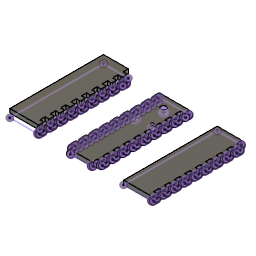
Motor Box (Autodesk Fusion 360 design; units mm, degrees)
part number: 2026-02-17-19-54-44-012
Autodesk Fusion 360 part; units mm, degrees
sketch "Sketch1" plane through (0, 0, 0) normal (0, 0, 1) x (1, 0, 0)
  line L0 (11.75, 48.5) -> (-11.75, 48.5)
  line L1 (-11.75, -48.5) -> (11.75, -48.5)
  line L2 (11.75, -48.5) -> (11.75, 48.5) construction
  line L3 (11.75, 48.5) -> (-11.75, -48.5) construction
  line L4 (-11.75, 48.5) -> (11.75, -48.5) construction
  line L5 (0, 48.5) -> (0, 37.3) construction
  circle A0 centre (0, 37.3) radius 2.7
  line L6 (1.85, 33.3) -> (-1.85, 33.3)
  line L7 (-1.85, 33.3) -> (-1.85, 41.3)
  line L8 (-1.85, 41.3) -> (1.85, 41.3)
  line L9 (1.85, 41.3) -> (1.85, 33.3)
  line L10 (1.85, 33.3) -> (-1.85, 41.3) construction
  line L11 (-1.85, 33.3) -> (1.85, 41.3) construction
  line L12 (0, 48.5) -> (0, 16.7) construction
  line L13 (0, 16.7) -> (8.75, 16.7) construction
  circle A1 centre (8.75, 16.7) radius 1.5
  circle A2 centre (-8.75, 16.7) radius 1.5
  line L14 (11.75, 48.5) -> (15.95, 48.5)
  line L15 (15.95, 48.5) -> (15.95, 43.1111)
  line L16 (15.95, 43.1111) -> (11.75, 43.1111)
  line L17 (11.75, 43.1111) -> (11.75, 37.7222)
  line L18 (11.75, 37.7222) -> (15.95, 37.7222)
  line L19 (15.95, 37.7222) -> (15.95, 32.3333)
  line L20 (15.95, 32.3333) -> (11.75, 32.3333)
  line L21 (11.75, 32.3333) -> (11.75, 26.9444)
  line L22 (11.75, 26.9444) -> (15.95, 26.9444)
  line L23 (15.95, 26.9444) -> (15.95, 21.5556)
  line L24 (15.95, 21.5556) -> (11.75, 21.5556)
  line L25 (11.75, 21.5556) -> (11.75, 16.1667)
  line L26 (11.75, 16.1667) -> (15.95, 16.1667)
  line L27 (15.95, 16.1667) -> (15.95, 10.7778)
  line L28 (15.95, 10.7778) -> (11.75, 10.7778)
  line L29 (11.75, 10.7778) -> (11.75, 5.3889)
  line L30 (11.75, 5.3889) -> (15.95, 5.3889)
  line L31 (15.95, 5.3889) -> (15.95, 0)
  line L32 (15.95, 0) -> (11.75, 0)
  line L33 (11.75, 0) -> (11.75, -5.3889)
  line L34 (11.75, -5.3889) -> (15.95, -5.3889)
  line L35 (15.95, -5.3889) -> (15.95, -10.7778)
  line L36 (15.95, -10.7778) -> (11.75, -10.7778)
  line L37 (11.75, -10.7778) -> (11.75, -16.1667)
  line L38 (11.75, -16.1667) -> (15.95, -16.1667)
  line L39 (15.95, -16.1667) -> (15.95, -21.5556)
  line L40 (15.95, -21.5556) -> (11.75, -21.5556)
  line L41 (11.75, -21.5556) -> (11.75, -26.9444)
  line L42 (11.75, -26.9444) -> (15.95, -26.9444)
  line L43 (15.95, -26.9444) -> (15.95, -32.3333)
  line L44 (15.95, -32.3333) -> (11.75, -32.3333)
  line L45 (11.75, -32.3333) -> (11.75, -37.7222)
  line L46 (11.75, -37.7222) -> (15.95, -37.7222)
  line L47 (15.95, -37.7222) -> (15.95, -43.1111)
  line L48 (15.95, -43.1111) -> (11.75, -43.1111)
  line L49 (11.75, -43.1111) -> (11.75, -48.5)
  line L50 (-15.95, 0) -> (-11.75, 0)
  line L51 (-15.95, 32.3333) -> (-11.75, 32.3333)
  line L52 (-15.95, -10.7778) -> (-11.75, -10.7778)
  line L53 (-15.95, 21.5556) -> (-11.75, 21.5556)
  line L54 (-11.75, 26.9444) -> (-15.95, 26.9444)
  line L55 (-15.95, -43.1111) -> (-11.75, -43.1111)
  line L56 (-15.95, -21.5556) -> (-11.75, -21.5556)
  line L57 (-15.95, -32.3333) -> (-11.75, -32.3333)
  line L58 (-11.75, -32.3333) -> (-11.75, -37.7222)
  line L59 (-15.95, 10.7778) -> (-11.75, 10.7778)
  line L60 (-11.75, 43.1111) -> (-11.75, 37.7222)
  line L61 (-15.95, 5.3889) -> (-15.95, 0)
  line L62 (-11.75, 10.7778) -> (-11.75, 5.3889)
  line L63 (-11.75, -48.5) -> (-11.75, 48.5) construction
  line L64 (-15.95, -16.1667) -> (-15.95, -21.5556)
  line L65 (-11.75, 21.5556) -> (-11.75, 16.1667)
  line L66 (-15.95, 48.5) -> (-15.95, 43.1111)
  line L67 (-15.95, 26.9444) -> (-15.95, 21.5556)
  line L68 (-15.95, -26.9444) -> (-15.95, -32.3333)
  line L69 (-11.75, 5.3889) -> (-15.95, 5.3889)
  line L70 (-11.75, -43.1111) -> (-11.75, -48.5)
  line L71 (-15.95, 16.1667) -> (-15.95, 10.7778)
  line L72 (-15.95, 37.7222) -> (-15.95, 32.3333)
  line L73 (-11.75, -26.9444) -> (-15.95, -26.9444)
  line L74 (-11.75, 32.3333) -> (-11.75, 26.9444)
  line L75 (-11.75, -5.3889) -> (-15.95, -5.3889)
  line L76 (-11.75, -10.7778) -> (-11.75, -16.1667)
  line L77 (-15.95, -37.7222) -> (-15.95, -43.1111)
  line L78 (-15.95, 43.1111) -> (-11.75, 43.1111)
  line L79 (-11.75, 16.1667) -> (-15.95, 16.1667)
  line L80 (-11.75, 0) -> (-11.75, -5.3889)
  line L81 (-15.95, -5.3889) -> (-15.95, -10.7778)
  line L82 (-11.75, -16.1667) -> (-15.95, -16.1667)
  line L83 (-11.75, -21.5556) -> (-11.75, -26.9444)
  line L84 (-11.75, -37.7222) -> (-15.95, -37.7222)
  line L85 (-11.75, 48.5) -> (-15.95, 48.5)
  line L86 (-11.75, 37.7222) -> (-15.95, 37.7222)
  point P0 (0, 37.3)
  dimension "d1" = 23.5
  dimension "d2" = 97
  dimension "d3" = 11.2
  dimension "d4" = 5.4
  dimension "d5" = 3.7
  dimension "d6" = 8
  dimension "d7" = 31.8
  dimension "d8" = 8.75
  dimension "d9" = 3
  dimension "d14" = 4.2
  dimension "d15" = 5.3889
  dimension "d16" = 5.3889
  dimension "d19" = 0
  dimension "d20" = -10.7778
  constraint horizontal L0
  constraint parallel L0 L1
  constraint coincident L3 origin
  constraint coincident L4 origin
  constraint midpoint L0 L5.start
  constraint perpendicular L0 L5
  constraint coincident P0 L5.end
  constraint horizontal L6
  constraint perpendicular L6 L7
  constraint parallel L6 L8
  constraint parallel L7 L9
  constraint coincident L10 P0
  constraint coincident L11 P0
  constraint perpendicular L6 L12
  constraint perpendicular L12 L13
  constraint coincident L13.end A1.centre
  constraint symmetric L12 A1 A2
  constraint horizontal L14
  constraint vertical L15
  constraint horizontal L16
  constraint perpendicular L16 L17
  constraint symmetric L0.start L12 L0.end
  constraint symmetric L1.end L12 L1.start
  constraint symmetric L12 L14.end L66.start
  constraint symmetric L12 L15.end L66.end
  constraint symmetric L12 L16.end L60.start
  constraint symmetric L12 L17.end L60.end
  constraint symmetric L12 L18.end L72.start
  constraint symmetric L12 L19.end L51.start
  constraint symmetric L12 L20.end L51.end
  constraint symmetric L12 L21.end L54.start
  constraint symmetric L12 L22.end L54.end
  constraint symmetric L12 L23.end L53.start
  constraint symmetric L12 L24.end L53.end
  constraint symmetric L12 L25.end L65.end
  constraint symmetric L12 L26.end L71.start
  constraint symmetric L12 L27.end L59.start
  constraint symmetric L12 L28.end L59.end
  constraint symmetric L12 L29.end L62.end
  constraint symmetric L12 L30.end L61.start
  constraint symmetric L12 L31.end L50.start
  constraint symmetric L12 L32.end L50.end
  constraint symmetric L12 L33.end L75.start
  constraint symmetric L12 L34.end L75.end
  constraint symmetric L12 L35.end L52.start
  constraint symmetric L12 L36.end L52.end
  constraint symmetric L12 L37.end L76.end
  constraint symmetric L12 L38.end L64.start
  constraint symmetric L12 L39.end L56.start
  constraint symmetric L12 L40.end L56.end
  constraint symmetric L12 L41.end L73.start
  constraint symmetric L12 L42.end L68.start
  constraint symmetric L12 L43.end L57.start
  constraint symmetric L12 L44.end L57.end
  constraint symmetric L12 L45.end L58.end
  constraint symmetric L12 L46.end L77.start
  constraint symmetric L12 L47.end L55.start
  constraint symmetric L12 L48.end L55.end
  constraint symmetric L12 L1.end L1.start
  constraint coincident L17.end L18.start
  measures "d1" distance of L1.start L1.end
  measures "d2" distance of L0.end L1.start
  measures "d3" distance of L5.start P0
  measures "d4" diameter of A0
  measures "d5" distance of L7.end L8.end
  measures "d6" distance of L6.end L7.end
  measures "d7" distance of L5.start L12.end
  measures "d8" distance of L12.end L13.end
  measures "d9" diameter of A1
  measures "d14" distance of L0.start L14.end
  measures "d15" distance of L0.start L16.end
  measures "d16" distance of L16.end L17.end
extrude "Extrude1" add sketch "Sketch1" along normal blind 4.2 contours L0 L1 L14 L15 L16 L17 L18 L19 L20 L21 L22 L23 L24 L25 L26 L27 L28 L29 L30 L31 L32 L33 L34 L35 L36 L37 L38 L39 L40 L41 L42 L43 L44 L45 L46 L47 L48 L49 L50 L51 L52 L53 L54 L55 L56 L57 L58 L59 L60 L61 L62 L64 L65 L66 L67 L68 L69 L70 L71 L72 L73 L74 L75 L76 L77 L78 L79 L80 L81 L82 L83 L84 L85 L86 | A0 L7 L8 L9 | A0 L6 L7 L9 makes body 1
sketch "Sketch2" plane through (15.95, 0, 0) normal (1, 0, 0) x (0, 1, 0)
  line L0 (-48.5, 0) -> (48.5, 0) construction
  line L1 (48.5, 0) -> (48.5, 30)
  line L2 (48.5, 30) -> (-48.5, 30)
  line L3 (-48.5, 30) -> (-48.5, 0)
  line L4 (-37.7222, 0) -> (-37.7222, 4.2)
  line L5 (-37.7222, 4.2) -> (-43.1111, 4.2)
  line L6 (-43.1111, 4.2) -> (-43.1111, 0)
  line L7 (-48.5, 0) -> (-43.1111, 0)
  line L8 (-37.7222, 0) -> (-32.3333, 0)
  line L9 (-32.3333, 4.2) -> (-32.3333, 0)
  line L10 (-26.9444, 4.2) -> (-32.3333, 4.2)
  line L11 (-26.9444, 0) -> (-26.9444, 4.2)
  line L12 (-26.9444, 0) -> (-21.5556, 0)
  line L13 (-21.5556, 4.2) -> (-21.5556, 0)
  line L14 (-16.1667, 4.2) -> (-21.5556, 4.2)
  line L15 (-16.1667, 0) -> (-16.1667, 4.2)
  line L16 (-16.1667, 0) -> (-10.7778, 0)
  line L17 (-10.7778, 4.2) -> (-10.7778, 0)
  line L18 (-5.3889, 4.2) -> (-10.7778, 4.2)
  line L19 (-5.3889, 0) -> (-5.3889, 4.2)
  line L20 (-5.3889, 0) -> (0, 0)
  line L21 (0, 4.2) -> (0, 0)
  line L22 (5.3889, 4.2) -> (0, 4.2)
  line L23 (5.3889, 0) -> (5.3889, 4.2)
  line L24 (5.3889, 0) -> (10.7778, 0)
  line L25 (10.7778, 4.2) -> (10.7778, 0)
  line L26 (16.1667, 4.2) -> (10.7778, 4.2)
  line L27 (16.1667, 0) -> (16.1667, 4.2)
  line L28 (16.1667, 0) -> (21.5556, 0)
  line L29 (21.5556, 4.2) -> (21.5556, 0)
  line L30 (26.9444, 4.2) -> (21.5556, 4.2)
  line L31 (26.9444, 0) -> (26.9444, 4.2)
  line L32 (26.9444, 0) -> (32.3333, 0)
  line L33 (32.3333, 4.2) -> (32.3333, 0)
  line L34 (37.7222, 4.2) -> (32.3333, 4.2)
  line L35 (37.7222, 0) -> (37.7222, 4.2)
  line L36 (37.7222, 0) -> (43.1111, 0)
  line L37 (43.1111, 4.2) -> (43.1111, 0)
  line L38 (48.5, 4.2) -> (43.1111, 4.2)
  line L39 (48.5, 0) -> (48.5, 4.2)
  point P0 (-48.5, 0)
  point P1 (-43.1111, 0)
  dimension "d23" = 97
  dimension "d24" = 30
  dimension "d25" = 5.3889
  dimension "d26" = 4.2
  dimension "d29" = 10.7778
  dimension "d30" = 0
  constraint horizontal L0
  constraint vertical L1
  constraint horizontal L2
  constraint vertical L3
  constraint coincident P0 L0.start
  constraint vertical L4
  constraint horizontal L5
  constraint vertical L6
  constraint coincident P1 L6.end
  measures "d23" distance of P0 L0.end
  measures "d24" distance of P0 L2.end
  measures "d25" distance of P1 L4.start
  measures "d26" distance of P1 L5.end
extrude "Extrude2" add sketch "Sketch2" against normal blind 4.2 separate body makes body 2
mirror "Mirror1" about plane through (0, 0, 0) normal (1, 0, 0) of bodies 2 makes body 3
move_body "Move1" bodies 3 to x (1, 0, 0) y (0, 1, 0) z (0, 0, 1) at (-29.0338, -1.4815, 0)
move_body "Move2" bodies 2 to x (1, 0, 0) y (0, 1, 0) z (0, 0, 1) at (32.2243, 4.8146, 0)
fillet "Fillet1" radius 1 38 edges at (-15.95, 48.5, 2.1) (-15.95, 43.1111, 2.1) (-15.95, 37.7222, 2.1) (-15.95, 32.3333, 2.1) (-15.95, 26.9444, 2.1) (-15.95, 21.5556, 2.1) (-15.95, 16.1667, 2.1) (-15.95, 10.7778, 2.1) (-15.95, 5.3889, 2.1) (-15.95, 0, 2.1) (-15.95, -5.3889, 2.1) (-15.95, -10.7778, 2.1) (-15.95, -16.1667, 2.1) (-15.95, -21.5556, 2.1) (-15.95, -26.9444, 2.1) (-15.95, -32.3333, 2.1) (-15.95, -37.7222, 2.1) (-15.95, -43.1111, 2.1) (15.95, -43.1111, 2.1) (15.95, -37.7222, 2.1) (15.95, -32.3333, 2.1) (15.95, -26.9444, 2.1) (15.95, -21.5556, 2.1) (15.95, -16.1667, 2.1) (15.95, -10.7778, 2.1) (15.95, -5.3889, 2.1) (11.75, -48.5, 2.1) (-11.75, -48.5, 2.1) (15.95, 0, 2.1) (15.95, 5.3889, 2.1) (15.95, 10.7778, 2.1) (15.95, 16.1667, 2.1) (15.95, 21.5556, 2.1) (15.95, 26.9444, 2.1) (15.95, 32.3333, 2.1) (15.95, 37.7222, 2.1) (15.95, 43.1111, 2.1) (15.95, 48.5, 2.1) on bodies 1
fillet "Fillet2" radius 1 19 edges at (46.0743, -43.6854, 0) (46.0743, -38.2965, 0) (46.0743, -32.9076, 0) (46.0743, -27.5187, 0) (46.0743, -22.1299, 0) (46.0743, -16.741, 0) (46.0743, -11.3521, 0) (46.0743, -5.9632, 0) (46.0743, -0.5743, 0) (46.0743, 4.8146, 0) (46.0743, 10.2035, 0) (46.0743, 15.5924, 0) (46.0743, 20.9813, 0) (46.0743, 26.3701, 0) (46.0743, 31.759, 0) (46.0743, 37.1479, 0) (46.0743, 42.5368, 0) (46.0743, 47.9257, 0) (46.0743, 53.3146, 4.2) on bodies 2
fillet "Fillet3" radius 1 18 edges at (-42.8838, -49.9815, 0) (-42.8838, -44.5926, 0) (-42.8838, -39.2037, 0) (-42.8838, -33.8149, 0) (-42.8838, -28.426, 0) (-42.8838, -23.0371, 0) (-42.8838, -17.6482, 0) (-42.8838, -12.2593, 0) (-42.8838, -6.8704, 0) (-42.8838, -1.4815, 0) (-42.8838, 3.9074, 0) (-42.8838, 9.2963, 0) (-42.8838, 14.6851, 0) (-42.8838, 20.074, 0) (-42.8838, 25.4629, 0) (-42.8838, 30.8518, 0) (-42.8838, 36.2407, 0) (-42.8838, 41.6296, 0) on bodies 3
move_body "Move3" bodies 3 to x (0, 0, 1) y (0, 1, 0) z (-1, 0, 0) at (-24.4783, 0, 65.4894)
move_body "Move4" bodies 3 to x (1, 0, 0) y (0, 1, 0) z (0, 0, 1) at (39.4783, 1.4815, -24.7055)
move_body "Move5" bodies 3 to x (1, 0, 0) y (0, 1, 0) z (0, 0, 1) at (-45.6208, -9.5411, 0)
move_body "Move6" bodies 2 to x (0, 0, 1) y (0, 1, 0) z (-1, 0, 0) at (69.5265, 0, -18.4221)
move_body "Move7" bodies 2 to x (1, 0, 0) y (0, 1, 0) z (0, 0, 1) at (-54.5265, -4.8146, -29.7522)
move_body "Move8" bodies 2 to x (1, 0, 0) y (0, 1, 0) z (0, 0, 1) at (59.8284, -15.152, 0)
move_body "Move9" bodies 3 to x (1, 0, 0) y (0, 1, 0) z (0, 0, 1) at (45.6208, 9.5411, 4.2)
move_body "Move10" bodies 3 to x (1, 0, 0) y (0, 1, 0) z (0, 0, 1) at (-45.2587, -4.9067, 0)
move_body "Move11" bodies 3 to x (1, 0, 0) y (0, 1, 0) z (0, 0, 1) at (-59.8284, 15.152, 4.2)
move_body "Move12" bodies 2 to x (1, 0, 0) y (0, 1, 0) z (0, 0, 1) at (-59.8284, 15.152, 4.2)
move_body "Move13" bodies 2 to x (1, 0, 0) y (0, 1, 0) z (0, 0, 1) at (59.2778, 0.0387, 0)
move_body "Move14" bodies 3 to x (1, 0, 0) y (0, 1, 0) z (0, 0, 1) at (45.2614, -9.0364, 0)
sketch "For Cutting" plane through (0, 0, 0) normal (0, 0, 1) x (1, 0, 0)
  arc A0 (70.0778, 47.5387) -> (69.0778, 48.5387) centre (69.0778, 47.5387) ccw
  line L0 (69.0778, 48.5387) -> (44.2778, 48.5387)
  line L1 (44.2778, 48.5387) -> (44.2778, -48.4613)
  line L2 (44.2778, -48.4613) -> (73.2778, -48.4613)
  arc A1 (73.2778, -48.4613) -> (74.2778, -47.4613) centre (73.2778, -47.4613) ccw
  line L3 (74.2778, -47.4613) -> (74.2778, -44.0724)
  arc A2 (74.2778, -44.0724) -> (73.2778, -43.0724) centre (73.2778, -44.0724) ccw
  line L4 (73.2778, -43.0724) -> (70.0778, -43.0724)
  line L5 (70.0778, -43.0724) -> (70.0778, -37.6835)
  line L6 (70.0778, -37.6835) -> (73.2778, -37.6835)
  arc A3 (73.2778, -37.6835) -> (74.2778, -36.6835) centre (73.2778, -36.6835) ccw
  line L7 (74.2778, -36.6835) -> (74.2778, -33.2946)
  arc A4 (74.2778, -33.2946) -> (73.2778, -32.2946) centre (73.2778, -33.2946) ccw
  line L8 (73.2778, -32.2946) -> (70.0778, -32.2946)
  line L9 (70.0778, -32.2946) -> (70.0778, -26.9057)
  line L10 (70.0778, -26.9057) -> (73.2778, -26.9057)
  arc A5 (73.2778, -26.9057) -> (74.2778, -25.9057) centre (73.2778, -25.9057) ccw
  line L11 (74.2778, -25.9057) -> (74.2778, -22.5168)
  arc A6 (74.2778, -22.5168) -> (73.2778, -21.5168) centre (73.2778, -22.5168) ccw
  line L12 (73.2778, -21.5168) -> (70.0778, -21.5168)
  line L13 (70.0778, -21.5168) -> (70.0778, -16.128)
  line L14 (70.0778, -16.128) -> (73.2778, -16.128)
  arc A7 (73.2778, -16.128) -> (74.2778, -15.128) centre (73.2778, -15.128) ccw
  line L15 (74.2778, -15.128) -> (74.2778, -11.7391)
  arc A8 (74.2778, -11.7391) -> (73.2778, -10.7391) centre (73.2778, -11.7391) ccw
  line L16 (73.2778, -10.7391) -> (70.0778, -10.7391)
  line L17 (70.0778, -10.7391) -> (70.0778, -5.3502)
  line L18 (70.0778, -5.3502) -> (73.2778, -5.3502)
  arc A9 (73.2778, -5.3502) -> (74.2778, -4.3502) centre (73.2778, -4.3502) ccw
  line L19 (74.2778, -4.3502) -> (74.2778, -0.9613)
  arc A10 (74.2778, -0.9613) -> (73.2778, 0.0387) centre (73.2778, -0.9613) ccw
  line L20 (73.2778, 0.0387) -> (70.0778, 0.0387)
  line L21 (70.0778, 0.0387) -> (70.0778, 5.4276)
  line L22 (70.0778, 5.4276) -> (73.2778, 5.4276)
  arc A11 (73.2778, 5.4276) -> (74.2778, 6.4276) centre (73.2778, 6.4276) ccw
  line L23 (74.2778, 6.4276) -> (74.2778, 9.8165)
  arc A12 (74.2778, 9.8165) -> (73.2778, 10.8165) centre (73.2778, 9.8165) ccw
  line L24 (73.2778, 10.8165) -> (70.0778, 10.8165)
  line L25 (70.0778, 10.8165) -> (70.0778, 16.2054)
  line L26 (70.0778, 16.2054) -> (73.2778, 16.2054)
  arc A13 (73.2778, 16.2054) -> (74.2778, 17.2054) centre (73.2778, 17.2054) ccw
  line L27 (74.2778, 17.2054) -> (74.2778, 20.5943)
  arc A14 (74.2778, 20.5943) -> (73.2778, 21.5943) centre (73.2778, 20.5943) ccw
  line L28 (73.2778, 21.5943) -> (70.0778, 21.5943)
  line L29 (70.0778, 21.5943) -> (70.0778, 26.9832)
  line L30 (70.0778, 26.9832) -> (73.2778, 26.9832)
  arc A15 (73.2778, 26.9832) -> (74.2778, 27.9832) centre (73.2778, 27.9832) ccw
  line L31 (74.2778, 27.9832) -> (74.2778, 31.372)
  arc A16 (74.2778, 31.372) -> (73.2778, 32.372) centre (73.2778, 31.372) ccw
  line L32 (73.2778, 32.372) -> (70.0778, 32.372)
  line L33 (70.0778, 32.372) -> (70.0778, 37.7609)
  line L34 (70.0778, 37.7609) -> (73.2778, 37.7609)
  arc A17 (73.2778, 37.7609) -> (74.2778, 38.7609) centre (73.2778, 38.7609) ccw
  line L35 (74.2778, 38.7609) -> (74.2778, 42.1498)
  arc A18 (74.2778, 42.1498) -> (73.2778, 43.1498) centre (73.2778, 42.1498) ccw
  line L36 (73.2778, 43.1498) -> (70.0778, 43.1498)
  line L37 (70.0778, 43.1498) -> (70.0778, 47.5387)
  arc A19 (15.95, 47.5) -> (14.95, 48.5) centre (14.95, 47.5) ccw
  line L38 (14.95, 48.5) -> (-14.95, 48.5)
  arc A20 (-14.95, 48.5) -> (-15.95, 47.5) centre (-14.95, 47.5) ccw
  line L39 (-15.95, 47.5) -> (-15.95, 44.1111)
  arc A21 (-15.95, 44.1111) -> (-14.95, 43.1111) centre (-14.95, 44.1111) ccw
  line L40 (-14.95, 43.1111) -> (-11.75, 43.1111)
  line L41 (-11.75, 43.1111) -> (-11.75, 37.7222)
  line L42 (-11.75, 37.7222) -> (-14.95, 37.7222)
  arc A22 (-14.95, 37.7222) -> (-15.95, 36.7222) centre (-14.95, 36.7222) ccw
  line L43 (-15.95, 36.7222) -> (-15.95, 33.3333)
  arc A23 (-15.95, 33.3333) -> (-14.95, 32.3333) centre (-14.95, 33.3333) ccw
  line L44 (-14.95, 32.3333) -> (-11.75, 32.3333)
  line L45 (-11.75, 32.3333) -> (-11.75, 26.9444)
  line L46 (-11.75, 26.9444) -> (-14.95, 26.9444)
  arc A24 (-14.95, 26.9444) -> (-15.95, 25.9444) centre (-14.95, 25.9444) ccw
  line L47 (-15.95, 25.9444) -> (-15.95, 22.5556)
  arc A25 (-15.95, 22.5556) -> (-14.95, 21.5556) centre (-14.95, 22.5556) ccw
  line L48 (-14.95, 21.5556) -> (-11.75, 21.5556)
  line L49 (-11.75, 21.5556) -> (-11.75, 16.1667)
  line L50 (-11.75, 16.1667) -> (-14.95, 16.1667)
  arc A26 (-14.95, 16.1667) -> (-15.95, 15.1667) centre (-14.95, 15.1667) ccw
  line L51 (-15.95, 15.1667) -> (-15.95, 11.7778)
  arc A27 (-15.95, 11.7778) -> (-14.95, 10.7778) centre (-14.95, 11.7778) ccw
  line L52 (-14.95, 10.7778) -> (-11.75, 10.7778)
  line L53 (-11.75, 10.7778) -> (-11.75, 5.3889)
  line L54 (-11.75, 5.3889) -> (-14.95, 5.3889)
  arc A28 (-14.95, 5.3889) -> (-15.95, 4.3889) centre (-14.95, 4.3889) ccw
  line L55 (-15.95, 4.3889) -> (-15.95, 1)
  arc A29 (-15.95, 1) -> (-14.95, 0) centre (-14.95, 1) ccw
  line L56 (-14.95, 0) -> (-11.75, 0)
  line L57 (-11.75, 0) -> (-11.75, -5.3889)
  line L58 (-11.75, -5.3889) -> (-14.95, -5.3889)
  arc A30 (-14.95, -5.3889) -> (-15.95, -6.3889) centre (-14.95, -6.3889) ccw
  line L59 (-15.95, -6.3889) -> (-15.95, -9.7778)
  arc A31 (-15.95, -9.7778) -> (-14.95, -10.7778) centre (-14.95, -9.7778) ccw
  line L60 (-14.95, -10.7778) -> (-11.75, -10.7778)
  line L61 (-11.75, -10.7778) -> (-11.75, -16.1667)
  line L62 (-11.75, -16.1667) -> (-14.95, -16.1667)
  arc A32 (-14.95, -16.1667) -> (-15.95, -17.1667) centre (-14.95, -17.1667) ccw
  line L63 (-15.95, -17.1667) -> (-15.95, -20.5556)
  arc A33 (-15.95, -20.5556) -> (-14.95, -21.5556) centre (-14.95, -20.5556) ccw
  line L64 (-14.95, -21.5556) -> (-11.75, -21.5556)
  line L65 (-11.75, -21.5556) -> (-11.75, -26.9444)
  line L66 (-11.75, -26.9444) -> (-14.95, -26.9444)
  arc A34 (-14.95, -26.9444) -> (-15.95, -27.9444) centre (-14.95, -27.9444) ccw
  line L67 (-15.95, -27.9444) -> (-15.95, -31.3333)
  arc A35 (-15.95, -31.3333) -> (-14.95, -32.3333) centre (-14.95, -31.3333) ccw
  line L68 (-14.95, -32.3333) -> (-11.75, -32.3333)
  line L69 (-11.75, -32.3333) -> (-11.75, -37.7222)
  line L70 (-11.75, -37.7222) -> (-14.95, -37.7222)
  arc A36 (-14.95, -37.7222) -> (-15.95, -38.7222) centre (-14.95, -38.7222) ccw
  line L71 (-15.95, -38.7222) -> (-15.95, -42.1111)
  arc A37 (-15.95, -42.1111) -> (-14.95, -43.1111) centre (-14.95, -42.1111) ccw
  line L72 (-14.95, -43.1111) -> (-11.75, -43.1111)
  line L73 (-11.75, -43.1111) -> (-11.75, -47.5)
  arc A38 (-11.75, -47.5) -> (-10.75, -48.5) centre (-10.75, -47.5) ccw
  line L74 (-10.75, -48.5) -> (10.75, -48.5)
  arc A39 (10.75, -48.5) -> (11.75, -47.5) centre (10.75, -47.5) ccw
  line L75 (11.75, -47.5) -> (11.75, -43.1111)
  line L76 (11.75, -43.1111) -> (14.95, -43.1111)
  arc A40 (14.95, -43.1111) -> (15.95, -42.1111) centre (14.95, -42.1111) ccw
  line L77 (15.95, -42.1111) -> (15.95, -38.7222)
  arc A41 (15.95, -38.7222) -> (14.95, -37.7222) centre (14.95, -38.7222) ccw
  line L78 (14.95, -37.7222) -> (11.75, -37.7222)
  line L79 (11.75, -37.7222) -> (11.75, -32.3333)
  line L80 (11.75, -32.3333) -> (14.95, -32.3333)
  arc A42 (14.95, -32.3333) -> (15.95, -31.3333) centre (14.95, -31.3333) ccw
  line L81 (15.95, -31.3333) -> (15.95, -27.9444)
  arc A43 (15.95, -27.9444) -> (14.95, -26.9444) centre (14.95, -27.9444) ccw
  line L82 (14.95, -26.9444) -> (11.75, -26.9444)
  line L83 (11.75, -26.9444) -> (11.75, -21.5556)
  line L84 (11.75, -21.5556) -> (14.95, -21.5556)
  arc A44 (14.95, -21.5556) -> (15.95, -20.5556) centre (14.95, -20.5556) ccw
  line L85 (15.95, -20.5556) -> (15.95, -17.1667)
  arc A45 (15.95, -17.1667) -> (14.95, -16.1667) centre (14.95, -17.1667) ccw
  line L86 (14.95, -16.1667) -> (11.75, -16.1667)
  line L87 (11.75, -16.1667) -> (11.75, -10.7778)
  line L88 (11.75, -10.7778) -> (14.95, -10.7778)
  arc A46 (14.95, -10.7778) -> (15.95, -9.7778) centre (14.95, -9.7778) ccw
  line L89 (15.95, -9.7778) -> (15.95, -6.3889)
  arc A47 (15.95, -6.3889) -> (14.95, -5.3889) centre (14.95, -6.3889) ccw
  line L90 (14.95, -5.3889) -> (11.75, -5.3889)
  line L91 (11.75, -5.3889) -> (11.75, 0)
  line L92 (11.75, 0) -> (14.95, 0)
  arc A48 (14.95, 0) -> (15.95, 1) centre (14.95, 1) ccw
  line L93 (15.95, 1) -> (15.95, 4.3889)
  arc A49 (15.95, 4.3889) -> (14.95, 5.3889) centre (14.95, 4.3889) ccw
  line L94 (14.95, 5.3889) -> (11.75, 5.3889)
  line L95 (11.75, 5.3889) -> (11.75, 10.7778)
  line L96 (11.75, 10.7778) -> (14.95, 10.7778)
  arc A50 (14.95, 10.7778) -> (15.95, 11.7778) centre (14.95, 11.7778) ccw
  line L97 (15.95, 11.7778) -> (15.95, 15.1667)
  arc A51 (15.95, 15.1667) -> (14.95, 16.1667) centre (14.95, 15.1667) ccw
  line L98 (14.95, 16.1667) -> (11.75, 16.1667)
  line L99 (11.75, 16.1667) -> (11.75, 21.5556)
  line L100 (11.75, 21.5556) -> (14.95, 21.5556)
  arc A52 (14.95, 21.5556) -> (15.95, 22.5556) centre (14.95, 22.5556) ccw
  line L101 (15.95, 22.5556) -> (15.95, 25.9444)
  arc A53 (15.95, 25.9444) -> (14.95, 26.9444) centre (14.95, 25.9444) ccw
  line L102 (14.95, 26.9444) -> (11.75, 26.9444)
  line L103 (11.75, 26.9444) -> (11.75, 32.3333)
  line L104 (11.75, 32.3333) -> (14.95, 32.3333)
  arc A54 (14.95, 32.3333) -> (15.95, 33.3333) centre (14.95, 33.3333) ccw
  line L105 (15.95, 33.3333) -> (15.95, 36.7222)
  arc A55 (15.95, 36.7222) -> (14.95, 37.7222) centre (14.95, 36.7222) ccw
  line L106 (14.95, 37.7222) -> (11.75, 37.7222)
  line L107 (11.75, 37.7222) -> (11.75, 43.1111)
  line L108 (11.75, 43.1111) -> (14.95, 43.1111)
  arc A56 (14.95, 43.1111) -> (15.95, 44.1111) centre (14.95, 44.1111) ccw
  line L109 (15.95, 44.1111) -> (15.95, 47.5)
  circle A57 centre (8.75, 16.7) radius 1.5
  circle A58 centre (0, 37.3) radius 2.7
  circle A59 centre (-8.75, 16.7) radius 1.5
  arc A60 (-44.8257, 43.32) -> (-45.8257, 44.32) centre (-45.8257, 43.32) ccw
  line L110 (-45.8257, 44.32) -> (-49.0257, 44.32)
  line L111 (-49.0257, 44.32) -> (-49.0257, 49.7089)
  line L112 (-49.0257, 49.7089) -> (-74.8257, 49.7089)
  line L113 (-74.8257, 49.7089) -> (-74.8257, -47.2911)
  line L114 (-74.8257, -47.2911) -> (-45.8257, -47.2911)
  arc A61 (-45.8257, -47.2911) -> (-44.8257, -46.2911) centre (-45.8257, -46.2911) ccw
  line L115 (-44.8257, -46.2911) -> (-44.8257, -42.9022)
  arc A62 (-44.8257, -42.9022) -> (-45.8257, -41.9022) centre (-45.8257, -42.9022) ccw
  line L116 (-45.8257, -41.9022) -> (-49.0257, -41.9022)
  line L117 (-49.0257, -41.9022) -> (-49.0257, -36.5133)
  line L118 (-49.0257, -36.5133) -> (-45.8257, -36.5133)
  arc A63 (-45.8257, -36.5133) -> (-44.8257, -35.5133) centre (-45.8257, -35.5133) ccw
  line L119 (-44.8257, -35.5133) -> (-44.8257, -32.1244)
  arc A64 (-44.8257, -32.1244) -> (-45.8257, -31.1244) centre (-45.8257, -32.1244) ccw
  line L120 (-45.8257, -31.1244) -> (-49.0257, -31.1244)
  line L121 (-49.0257, -31.1244) -> (-49.0257, -25.7355)
  line L122 (-49.0257, -25.7355) -> (-45.8257, -25.7355)
  arc A65 (-45.8257, -25.7355) -> (-44.8257, -24.7355) centre (-45.8257, -24.7355) ccw
  line L123 (-44.8257, -24.7355) -> (-44.8257, -21.3466)
  arc A66 (-44.8257, -21.3466) -> (-45.8257, -20.3466) centre (-45.8257, -21.3466) ccw
  line L124 (-45.8257, -20.3466) -> (-49.0257, -20.3466)
  line L125 (-49.0257, -20.3466) -> (-49.0257, -14.9577)
  line L126 (-49.0257, -14.9577) -> (-45.8257, -14.9577)
  arc A67 (-45.8257, -14.9577) -> (-44.8257, -13.9577) centre (-45.8257, -13.9577) ccw
  line L127 (-44.8257, -13.9577) -> (-44.8257, -10.5689)
  arc A68 (-44.8257, -10.5689) -> (-45.8257, -9.5689) centre (-45.8257, -10.5689) ccw
  line L128 (-45.8257, -9.5689) -> (-49.0257, -9.5689)
  line L129 (-49.0257, -9.5689) -> (-49.0257, -4.18)
  line L130 (-49.0257, -4.18) -> (-45.8257, -4.18)
  arc A69 (-45.8257, -4.18) -> (-44.8257, -3.18) centre (-45.8257, -3.18) ccw
  line L131 (-44.8257, -3.18) -> (-44.8257, 0.2089)
  arc A70 (-44.8257, 0.2089) -> (-45.8257, 1.2089) centre (-45.8257, 0.2089) ccw
  line L132 (-45.8257, 1.2089) -> (-49.0257, 1.2089)
  line L133 (-49.0257, 1.2089) -> (-49.0257, 6.5978)
  line L134 (-49.0257, 6.5978) -> (-45.8257, 6.5978)
  arc A71 (-45.8257, 6.5978) -> (-44.8257, 7.5978) centre (-45.8257, 7.5978) ccw
  line L135 (-44.8257, 7.5978) -> (-44.8257, 10.9867)
  arc A72 (-44.8257, 10.9867) -> (-45.8257, 11.9867) centre (-45.8257, 10.9867) ccw
  line L136 (-45.8257, 11.9867) -> (-49.0257, 11.9867)
  line L137 (-49.0257, 11.9867) -> (-49.0257, 17.3756)
  line L138 (-49.0257, 17.3756) -> (-45.8257, 17.3756)
  arc A73 (-45.8257, 17.3756) -> (-44.8257, 18.3756) centre (-45.8257, 18.3756) ccw
  line L139 (-44.8257, 18.3756) -> (-44.8257, 21.7645)
  arc A74 (-44.8257, 21.7645) -> (-45.8257, 22.7645) centre (-45.8257, 21.7645) ccw
  line L140 (-45.8257, 22.7645) -> (-49.0257, 22.7645)
  line L141 (-49.0257, 22.7645) -> (-49.0257, 28.1534)
  line L142 (-49.0257, 28.1534) -> (-45.8257, 28.1534)
  arc A75 (-45.8257, 28.1534) -> (-44.8257, 29.1534) centre (-45.8257, 29.1534) ccw
  line L143 (-44.8257, 29.1534) -> (-44.8257, 32.5423)
  arc A76 (-44.8257, 32.5423) -> (-45.8257, 33.5423) centre (-45.8257, 32.5423) ccw
  line L144 (-45.8257, 33.5423) -> (-49.0257, 33.5423)
  line L145 (-49.0257, 33.5423) -> (-49.0257, 38.9311)
  line L146 (-49.0257, 38.9311) -> (-45.8257, 38.9311)
  arc A77 (-45.8257, 38.9311) -> (-44.8257, 39.9311) centre (-45.8257, 39.9311) ccw
  line L147 (-44.8257, 39.9311) -> (-44.8257, 43.32)
equation "d2 = length"
equation "d8 = ( 17.5 / 2 ) * 1 mm"
equation "num_teeth = 9"
equation "thickness = 4.2 mm"
equation "length = 97 mm"
equation "d14 = thickness"
equation "d15 = length / ( 2 * num_teeth )"
equation "d16 = length / ( 2 * num_teeth )"
equation "d18 = num_teeth"
equation "d20 = -1 * length / num_teeth"
equation "d21 = thickness"
equation "d23 = length"
equation "d25 = length / ( num_teeth * 2 )"
equation "d26 = thickness"
equation "d27 = num_teeth"
equation "d29 = length / num_teeth"
equation "d31 = -thickness"
named bodies: "Bottom", "Right", "Left"
